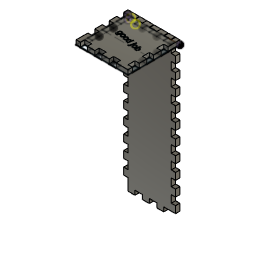
laser cut led  v7 (Autodesk Fusion 360 design; units mm, degrees)
Autodesk Fusion 360 part; units mm, degrees
sketch "Sketch1" plane through (0, 0, 0) normal (0, 1, 0) x (1, 0, 0)
  line L0 (0, 0) -> (30, 0)
  line L1 (30, 0) -> (30, -100)
  line L2 (30, -100) -> (0, -100)
  line L3 (0, -100) -> (0, 0)
  line L4 (0, 0) -> (4.8, 0)
  line L5 (4.8, 0) -> (4.8, 3)
  line L6 (4.8, 3) -> (0, 3)
  line L7 (0, 3) -> (0, 0)
  line L8 (4.8, 3) -> (10, 3) construction
  line L9 (10, 3) -> (14.8, 3)
  line L10 (14.8, 3) -> (14.8, 0)
  line L11 (14.8, 0) -> (10, 0)
  line L12 (10, 0) -> (10, 3)
  line L13 (14.8, 3) -> (20, 3) construction
  line L14 (20, 3) -> (24.8, 3)
  line L15 (24.8, 3) -> (24.8, 0)
  line L16 (24.8, 0) -> (20, 0)
  line L17 (20, 0) -> (20, 3)
  line L18 (0, -50) -> (30, -50) construction
  line L19 (30, 0) -> (33, 0)
  line L20 (33, 0) -> (33, -4.8)
  line L21 (33, -4.8) -> (30, -4.8)
  line L22 (30, -4.8) -> (30, 0)
  line L23 (33, -4.8) -> (33, -10) construction
  line L24 (33, -14.8) -> (30, -14.8)
  line L25 (30, -14.8) -> (30, -10)
  line L26 (33, -10) -> (33, -14.8)
  line L27 (30, -10) -> (33, -10)
  line L28 (33, -14.8) -> (33, -20) construction
  line L29 (33, -24.8) -> (30, -24.8)
  line L30 (30, -24.8) -> (30, -20)
  line L31 (33, -20) -> (33, -24.8)
  line L32 (30, -20) -> (33, -20)
  line L33 (33, -24.8) -> (33, -30) construction
  line L34 (33, -34.8) -> (30, -34.8)
  line L35 (30, -34.8) -> (30, -30)
  line L36 (33, -30) -> (33, -34.8)
  line L37 (30, -30) -> (33, -30)
  line L38 (33, -34.8) -> (33, -40) construction
  line L39 (33, -44.8) -> (30, -44.8)
  line L40 (30, -44.8) -> (30, -40)
  line L41 (33, -40) -> (33, -44.8)
  line L42 (30, -40) -> (33, -40)
  line L43 (33, -44.8) -> (33, -50) construction
  line L44 (33, -54.8) -> (30, -54.8)
  line L45 (30, -54.8) -> (30, -50)
  line L46 (33, -50) -> (33, -54.8)
  line L47 (30, -50) -> (33, -50)
  line L48 (33, -54.8) -> (33, -60) construction
  line L49 (33, -64.8) -> (30, -64.8)
  line L50 (30, -64.8) -> (30, -60)
  line L51 (33, -60) -> (33, -64.8)
  line L52 (30, -60) -> (33, -60)
  line L53 (33, -64.8) -> (33, -70) construction
  line L54 (33, -74.8) -> (30, -74.8)
  line L55 (30, -74.8) -> (30, -70)
  line L56 (33, -70) -> (33, -74.8)
  line L57 (30, -70) -> (33, -70)
  line L58 (33, -74.8) -> (33, -80) construction
  line L59 (33, -84.8) -> (30, -84.8)
  line L60 (30, -84.8) -> (30, -80)
  line L61 (33, -80) -> (33, -84.8)
  line L62 (30, -80) -> (33, -80)
  line L63 (33, -84.8) -> (33, -90) construction
  line L64 (33, -94.8) -> (30, -94.8)
  line L65 (30, -94.8) -> (30, -90)
  line L66 (33, -90) -> (33, -94.8)
  line L67 (30, -90) -> (33, -90)
  line L68 (33, -94.8) -> (33, -100) construction
  line L69 (-3, -100) -> (-3, -95.2)
  line L70 (-3, -95.2) -> (0, -95.2)
  line L71 (0, -95.2) -> (0, -100)
  line L72 (-3, -100) -> (0, -100)
  line L73 (-3, -95.2) -> (-3, -90) construction
  line L74 (0, -85.2) -> (0, -90)
  line L75 (-3, -85.2) -> (0, -85.2)
  line L76 (-3, -90) -> (-3, -85.2)
  line L77 (-3, -90) -> (0, -90)
  line L78 (-3, -85.2) -> (-3, -80) construction
  line L79 (0, -75.2) -> (0, -80)
  line L80 (-3, -75.2) -> (0, -75.2)
  line L81 (-3, -80) -> (-3, -75.2)
  line L82 (-3, -80) -> (0, -80)
  line L83 (-3, -75.2) -> (-3, -70) construction
  line L84 (0, -65.2) -> (0, -70)
  line L85 (-3, -65.2) -> (0, -65.2)
  line L86 (-3, -70) -> (-3, -65.2)
  line L87 (-3, -70) -> (0, -70)
  line L88 (-3, -65.2) -> (-3, -60) construction
  line L89 (0, -55.2) -> (0, -60)
  line L90 (-3, -55.2) -> (0, -55.2)
  line L91 (-3, -60) -> (-3, -55.2)
  line L92 (-3, -60) -> (0, -60)
  line L93 (-3, -55.2) -> (-3, -50) construction
  line L94 (0, -45.2) -> (0, -50)
  line L95 (-3, -45.2) -> (0, -45.2)
  line L96 (-3, -50) -> (-3, -45.2)
  line L97 (-3, -50) -> (0, -50)
  line L98 (-3, -45.2) -> (-3, -40) construction
  line L99 (0, -35.2) -> (0, -40)
  line L100 (-3, -35.2) -> (0, -35.2)
  line L101 (-3, -40) -> (-3, -35.2)
  line L102 (-3, -40) -> (0, -40)
  line L103 (-3, -35.2) -> (-3, -30) construction
  line L104 (0, -25.2) -> (0, -30)
  line L105 (-3, -25.2) -> (0, -25.2)
  line L106 (-3, -30) -> (-3, -25.2)
  line L107 (-3, -30) -> (0, -30)
  line L108 (-3, -25.2) -> (-3, -20) construction
  line L109 (0, -15.2) -> (0, -20)
  line L110 (-3, -15.2) -> (0, -15.2)
  line L111 (-3, -20) -> (-3, -15.2)
  line L112 (-3, -20) -> (0, -20)
  line L113 (-3, -15.2) -> (-3, -10) construction
  line L114 (0, -5.2) -> (0, -10)
  line L115 (-3, -5.2) -> (0, -5.2)
  line L116 (-3, -10) -> (-3, -5.2)
  line L117 (-3, -10) -> (0, -10)
  line L118 (-3, -5.2) -> (-3, 0) construction
  line L119 (30, -100) -> (25.2, -100)
  line L120 (25.2, -100) -> (25.2, -103)
  line L121 (25.2, -103) -> (30, -103)
  line L122 (30, -103) -> (30, -100)
  line L123 (25.2, -103) -> (20, -103) construction
  line L124 (15.2, -100) -> (15.2, -103)
  line L125 (15.2, -103) -> (10, -103) construction
  line L126 (20, -103) -> (20, -100)
  line L127 (15.2, -103) -> (20, -103)
  line L128 (20, -100) -> (15.2, -100)
  line L129 (5.2, -100) -> (5.2, -103)
  line L130 (5.2, -103) -> (0, -103) construction
  line L131 (10, -103) -> (10, -100)
  line L132 (5.2, -103) -> (10, -103)
  line L133 (10, -100) -> (5.2, -100)
  point P0 (0, -90)
  point P1 (0, -80)
  point P2 (0, -70)
  point P3 (0, -60)
  point P4 (0, -50)
  point P5 (0, -40)
  point P6 (0, -30)
  point P7 (0, -20)
  point P8 (0, -10)
  dimension "d1" = 30
  dimension "d2" = 100
  dimension "d8" = 4.8
  dimension "d9" = 3
  dimension "d12" = 4.8
  dimension "d13" = 3
  dimension "d15" = 5.2
  dimension "d16" = 5.2
  dimension "d17" = 4.8
  dimension "d18" = 3
  dimension "d20" = 3
  dimension "d21" = 4.8
  dimension "d22" = 5.2
  dimension "d25" = 0
  dimension "d26" = -90
  dimension "d27" = 3
  dimension "d28" = 4.8
  dimension "d29" = 5.2
  dimension "d32" = 0
  dimension "d33" = 90
  dimension "d34" = 4.8
  dimension "d35" = 3
  dimension "d36" = 5.2
  dimension "d40" = -20
  dimension "d41" = 0
  constraint horizontal L0
  constraint vertical L1
  constraint vertical L3
  constraint coincident L0.start L3.end
  constraint horizontal L4
  constraint vertical L5
  constraint horizontal L6
  constraint vertical L7
  constraint perpendicular L5 L8
  constraint horizontal L9
  constraint vertical L10
  constraint horizontal L11
  constraint vertical L12
  constraint coincident L5.end L6.start
  constraint perpendicular L10 L13
  constraint horizontal L14
  constraint vertical L15
  constraint horizontal L16
  constraint vertical L17
  constraint midpoint L3 P4
  constraint midpoint L1 L18.end
  constraint horizontal L19
  constraint vertical L20
  constraint horizontal L21
  constraint vertical L22
  constraint perpendicular L21 L23
  constraint vertical L69
  constraint horizontal L70
  constraint vertical L71
  constraint parallel L2 L64
  constraint equal L70 L72
  constraint coincident L2.end L3.start
  constraint perpendicular L70 L73
  constraint horizontal L119
  constraint vertical L120
  constraint horizontal L121
  constraint vertical L122
  constraint perpendicular L120 L123
  measures "d1" distance of L0.start L0.end
  measures "d2" distance of L0.start L2.end
  measures "d8" distance of L0.start L4.end
  measures "d9" distance of L0.start L6.end
  measures "d12" distance of L8.end L9.end
  measures "d13" distance of L8.end L11.end
  measures "d15" distance of L5.end L8.end
  measures "d16" distance of L9.end L13.end
  measures "d17" distance of L13.end L14.end
  measures "d18" distance of L13.end L16.end
  measures "d20" distance of L0.end L19.end
  measures "d21" distance of L0.end L21.end
  measures "d22" distance of L20.end L23.end
  measures "d27" distance of L2.end L69.start
  measures "d28" distance of L2.end L70.end
  measures "d29" distance of L69.end L73.end
  measures "d34" distance of L1.end L119.end
  measures "d35" distance of L1.end L121.end
  measures "d36" distance of L120.end L123.end
extrude "Extrude1" add sketch "Sketch1" along normal blind 3 makes body 1
sketch "Sketch2" plane through (0, 0, 100) normal (0, 0, 1) x (-1, 0, 0)
  line L0 (0, 0) -> (-5.2, 0) construction
  line L1 (0, -2) -> (0, 0) construction
  line L2 (3, -3) -> (-33, -3)
  line L3 (-33, -3) -> (-33, 33)
  line L4 (-33, 33) -> (3, 33)
  line L5 (3, 33) -> (3, -3)
  line L6 (3, 0) -> (0, 0)
  line L7 (0, 0) -> (0, 4.8)
  line L8 (0, 4.8) -> (3, 4.8)
  line L9 (3, 4.8) -> (3, 0)
  line L10 (0, 4.8) -> (0, 10) construction
  line L11 (3, 10) -> (0, 10)
  line L12 (0, 10) -> (0, 14.8)
  line L13 (0, 14.8) -> (3, 14.8)
  line L14 (0, 14.8) -> (0, 20) construction
  line L15 (3, 14.8) -> (3, 10)
  line L16 (3, 20) -> (0, 20)
  line L17 (0, 20) -> (0, 24.8)
  line L18 (0, 24.8) -> (3, 24.8)
  line L19 (0, 24.8) -> (0, 30) construction
  line L20 (3, 24.8) -> (3, 20)
  line L21 (0, 30) -> (-4.8, 30)
  line L22 (-4.8, 30) -> (-4.8, 33)
  line L23 (-4.8, 33) -> (0, 33)
  line L24 (0, 33) -> (0, 30)
  line L25 (-4.8, 30) -> (-10, 30) construction
  line L26 (-14.8, 33) -> (-10, 33)
  line L27 (-14.8, 30) -> (-20, 30) construction
  line L28 (-10, 30) -> (-14.8, 30)
  line L29 (-10, 33) -> (-10, 30)
  line L30 (-14.8, 30) -> (-14.8, 33)
  line L31 (-24.8, 33) -> (-20, 33)
  line L32 (-24.8, 30) -> (-30, 30) construction
  line L33 (-20, 30) -> (-24.8, 30)
  line L34 (-20, 33) -> (-20, 30)
  line L35 (-24.8, 30) -> (-24.8, 33)
  line L36 (-30, 30) -> (-33, 30)
  line L37 (-33, 30) -> (-33, 25.2)
  line L38 (-33, 25.2) -> (-30, 25.2)
  line L39 (-30, 25.2) -> (-30, 30)
  line L40 (-30, 25.2) -> (-30, 20) construction
  line L41 (-30, 15.2) -> (-30, 20)
  line L42 (-30, 20) -> (-33, 20)
  line L43 (-33, 15.2) -> (-30, 15.2)
  line L44 (-33, 20) -> (-33, 15.2)
  line L45 (-30, 15.2) -> (-30, 10) construction
  line L46 (-30, 5.2) -> (-30, 10)
  line L47 (-30, 10) -> (-33, 10)
  line L48 (-33, 5.2) -> (-30, 5.2)
  line L49 (-33, 10) -> (-33, 5.2)
  line L50 (-30, 5.2) -> (-30, 0) construction
  line L51 (3, 15) -> (-33, 15) construction
  line L52 (-10, 0) -> (-14.8, 0) construction
  line L53 (-14.8, 0) -> (-14.8, -3)
  line L54 (-14.8, 0) -> (-20, 0)
  line L55 (-24.8, 0) -> (-24.8, -3)
  line L56 (-4.8, 0) -> (-10, 0)
  line L57 (-4.8, 0) -> (-4.8, -3)
  line L58 (0, -3) -> (0, 0) construction
  line L59 (0, 0) -> (-4.8, 0) construction
  line L60 (-10, -3) -> (-10, 0)
  line L61 (-20, -3) -> (-20, 0)
  line L62 (-20, 0) -> (-24.8, 0) construction
  line L63 (-4.8, -3) -> (0, -3)
  line L64 (-24.8, -3) -> (-20, -3)
  line L65 (-14.8, -3) -> (-10, -3)
  line L66 (-24.8, 0) -> (-29.6, 0)
  line L67 (-29.6, 0) -> (-29.6, -3)
  line L68 (-29.6, -3) -> (-24.8, -3) construction
  line L69 (-24.8, -3) -> (-24.8, 0) construction
  point P0 (3, -3)
  point P1 (-33, -3)
  point P2 (0, 10)
  point P3 (0, 10)
  point P4 (0, 20)
  point P5 (0, 20)
  dimension "d44" = 36
  dimension "d51" = 3
  dimension "d52" = 4.8
  dimension "d53" = 5.2
  dimension "d56" = 0
  dimension "d57" = 20
  dimension "d75" = 4.8
  dimension "d76" = 3
  dimension "d77" = 5.2
  dimension "d80" = -20
  dimension "d81" = 0
  dimension "d84" = 36
  dimension "d85" = 3
  dimension "d86" = 4.8
  dimension "d87" = 5.2
  dimension "d90" = 0
  dimension "d91" = -20
  dimension "d108" = 33
  dimension "d109" = 4.8
  constraint horizontal L2
  constraint horizontal L4
  constraint vertical L5
  constraint coincident P0 L2.start
  constraint coincident P1 L2.end
  constraint horizontal L6
  constraint vertical L7
  constraint horizontal L8
  constraint vertical L9
  constraint coincident L5 L6.start
  constraint perpendicular L8 L10
  constraint coincident L0.start L1.end
  constraint horizontal L21
  constraint vertical L22
  constraint horizontal L23
  constraint vertical L24
  constraint perpendicular L22 L25
  constraint horizontal L36
  constraint vertical L37
  constraint horizontal L38
  constraint vertical L39
  constraint perpendicular L38 L40
  constraint midpoint L5 L51.start
  constraint midpoint L3 L51.end
  constraint symmetric L19.end L51 L0.start
  constraint symmetric L21.end L51 L56.start
  constraint symmetric L22.end L51 L57.end
  constraint symmetric L23.end L51 L58.start
  constraint symmetric L25.end L51 L52.start
  constraint symmetric L26.start L51 L53.end
  constraint symmetric L26.end L51 L60.start
  constraint symmetric L27.start L51 L52.end
  constraint symmetric L27.end L51 L54.end
  constraint symmetric L31.start L51 L55.end
  constraint symmetric L31.end L51 L61.start
  constraint symmetric L32.start L51 L55.start
  constraint horizontal L66
  constraint vertical L67
  constraint horizontal L68
  constraint vertical L69
  measures "d44" distance of P1 L3.end
  measures "d51" distance of L6.start L0.start
  measures "d52" distance of L6.start L8.end
  measures "d53" distance of L7.end P3
  measures "d75" distance of L19.end L21.end
  measures "d76" distance of L19.end L23.end
  measures "d77" distance of L21.end L25.end
  measures "d84" distance of L3.end L4.end
  measures "d85" distance of L32.end L36.end
  measures "d86" distance of L32.end L38.end
  measures "d87" distance of L38.end L40.end
  measures "d108" distance of L4 L50.end
  measures "d109" distance of L55.start L66.end
extrude "Extrude4" add sketch "Sketch2" along normal blind 3 separate body contours L2 L3 L4 L5 L6 L7 L8 L11 L12 L13 L16 L17 L18 L21 L22 L24 L28 L29 L30 L33 L34 L35 L36 L38 L39 L41 L42 L43 L46 L47 L48 L53 L54 L55 L56 L57 L60 L61 L63 L64 L65 L66 L67 | L2 L56 L57 L60 | L2 L53 L54 L61 | L2 L55 L66 L67 makes body 2
sketch "Sketch3" plane through (0, 0, 103) normal (0, 0, 1) x (-1, 0, 0)
  line L0 (-33, -3) -> (3, -3)
  line L1 (3, -3) -> (3, 0)
  line L2 (3, 0) -> (0, 0)
  line L3 (0, 0) -> (0, 4.8)
  line L4 (0, 4.8) -> (3, 4.8)
  line L5 (3, 4.8) -> (3, 10)
  line L6 (3, 10) -> (0, 10)
  line L7 (0, 10) -> (0, 14.8)
  line L8 (0, 14.8) -> (3, 14.8)
  line L9 (3, 14.8) -> (3, 20)
  line L10 (3, 20) -> (0, 20)
  line L11 (0, 20) -> (0, 24.8)
  line L12 (0, 24.8) -> (3, 24.8)
  line L13 (3, 24.8) -> (3, 33)
  line L14 (3, 33) -> (0, 33)
  line L15 (0, 33) -> (0, 30)
  line L16 (0, 30) -> (-4.8, 30)
  line L17 (-4.8, 30) -> (-4.8, 33)
  line L18 (-4.8, 33) -> (-10, 33)
  line L19 (-10, 33) -> (-10, 30)
  line L20 (-10, 30) -> (-14.8, 30)
  line L21 (-14.8, 30) -> (-14.8, 33)
  line L22 (-14.8, 33) -> (-20, 33)
  line L23 (-20, 33) -> (-20, 30)
  line L24 (-20, 30) -> (-24.8, 30)
  line L25 (-24.8, 30) -> (-24.8, 33)
  line L26 (-24.8, 33) -> (-33, 33)
  line L27 (-33, 33) -> (-33, 30)
  line L28 (-33, 30) -> (-30, 30)
  line L29 (-30, 30) -> (-30, 25.2)
  line L30 (-30, 25.2) -> (-33, 25.2)
  line L31 (-33, 25.2) -> (-33, 20)
  line L32 (-33, 20) -> (-30, 20)
  line L33 (-30, 20) -> (-30, 15.2)
  line L34 (-30, 15.2) -> (-33, 15.2)
  line L35 (-33, 15.2) -> (-33, 10)
  line L36 (-33, 10) -> (-30, 10)
  line L37 (-30, 10) -> (-30, 5.2)
  line L38 (-30, 5.2) -> (-33, 5.2)
  line L39 (-33, 5.2) -> (-33, -3)
  line L40 (-6.1133, 15.5844) -> (-20.7441, 18.8917) construction
  line L41 (-20.7441, 18.8917) -> (-21.8466, 14.0148) construction
  line L42 (-21.8466, 14.0148) -> (-7.2157, 10.7074) construction
  line L43 (-7.2157, 10.7074) -> (-6.1133, 15.5844) construction
  line L44 (-14.5311, 12.3611) -> (-17.9487, -2.7575) construction
  line L45 (-21.2953, 16.4532) -> (-33, 19.0991) construction
  dimension "d97" = 5
  dimension "d98" = 15
  dimension "d106" = 15.5
  dimension "d107" = 12
  text T0 "good job" font "Arial" height 5 align ink ink in box 0 x 0 at (-6.1133, 15.5844) x (-0.975389, 0.220489) y (-0.220489, -0.975389) spacing 1 kerned height is em
  constraint perpendicular L40 L41
  constraint parallel L40 L42
  constraint parallel L41 L43
  constraint midpoint L42 L44.start
  constraint perpendicular L42 L44
  constraint midpoint L41 L45.start
  constraint perpendicular L41 L45
  constraint coincident L35 L45.end
  measures "d97" distance of L40.start L42.end
  measures "d98" distance of L41.end L42.end
  measures "d106" distance of L44.start L44.end
  measures "d107" distance of L45.start L45.end
extrude "Extrude5" cut sketch "Sketch3" against normal blind 1 text T0 bodies 2
sketch "TOP_DXF" plane through (0, 0, 103) normal (0, 0, 1) x (-1, 0, 0)
  spline S0 degree 3 poles (-10.2517, 15.4704) (-10.0879, 15.4205) (-9.7707, 15.3239) (-9.5682, 15.0623) (-9.4702, 14.9358) knots 0 0 0 0 0.049993 0.096791 0.096791 0.096791 0.096791
  spline S1 degree 3 poles (-9.4702, 14.9358) (-9.4051, 14.7805) (-9.263, 14.4413) (-9.3289, 14.0777) (-9.3646, 13.8807) knots 0 0 0 0 0.049486 0.108074 0.108074 0.108074 0.108074
  spline S2 degree 3 poles (-9.3646, 13.8807) (-9.4225, 13.67) (-9.5289, 13.2826) (-9.8458, 13.0393) (-9.9903, 12.9283) knots 0 0 0 0 0.063477 0.116753 0.116753 0.116753 0.116753
  spline S3 degree 3 poles (-9.9903, 12.9283) (-10.1253, 12.8727) (-10.4018, 12.7588) (-10.6978, 12.804) (-10.8492, 12.8271) knots 0 0 0 0 0.042941 0.087955 0.087955 0.087955 0.087955
  spline S4 degree 3 poles (-10.8492, 12.8271) (-11.0107, 12.877) (-11.3256, 12.9742) (-11.5266, 13.2347) (-11.6245, 13.3615) knots 0 0 0 0 0.049367 0.096242 0.096242 0.096242 0.096242
  spline S5 degree 3 poles (-11.6245, 13.3615) (-11.6914, 13.514) (-11.8346, 13.8403) (-11.7742, 14.1928) (-11.7421, 14.3806) knots 0 0 0 0 0.048869 0.104602 0.104602 0.104602 0.104602
  spline S6 degree 3 poles (-11.7421, 14.3806) (-11.7059, 14.5272) (-11.6409, 14.791) (-11.4893, 15.0157) (-11.422, 15.1154) knots 0 0 0 0 0.044866 0.080708 0.080708 0.080708 0.080708
  spline S7 degree 3 poles (-11.422, 15.1154) (-11.3476, 15.1913) (-11.1982, 15.3434) (-10.9979, 15.4168) (-10.8975, 15.4537) knots 0 0 0 0 0.03145 0.063109 0.063109 0.063109 0.063109
  spline S8 degree 3 poles (-10.8975, 15.4537) (-10.7914, 15.4771) (-10.5773, 15.5245) (-10.3609, 15.4885) (-10.2517, 15.4704) knots 0 0 0 0 0.032274 0.065137 0.065137 0.065137 0.065137
  line L0 (-17.4905, 13.3773) -> (-16.7013, 16.8683)
  line L1 (-16.7013, 16.8683) -> (-16.3037, 16.7784)
  line L2 (-16.3037, 16.7784) -> (-16.3758, 16.4593)
  spline S9 degree 3 poles (-16.3758, 16.4593) (-16.2604, 16.5485) (-16.0264, 16.7294) (-15.7324, 16.6937) (-15.5835, 16.6756) knots 0 0 0 0 0.042007 0.085152 0.085152 0.085152 0.085152
  spline S10 degree 3 poles (-15.5835, 16.6756) (-15.4862, 16.6463) (-15.2916, 16.5877) (-15.1407, 16.4514) (-15.0651, 16.3833) knots 0 0 0 0 0.03006 0.060176 0.060176 0.060176 0.060176
  spline S11 degree 3 poles (-15.0651, 16.3833) (-14.9989, 16.303) (-14.8635, 16.1389) (-14.8066, 15.9337) (-14.7775, 15.8289) knots 0 0 0 0 0.030848 0.063081 0.063081 0.063081 0.063081
  spline S12 degree 3 poles (-14.7775, 15.8289) (-14.7608, 15.7139) (-14.7259, 15.4736) (-14.7703, 15.2348) (-14.7934, 15.1104) knots 0 0 0 0 0.034627 0.072303 0.072303 0.072303 0.072303
  spline S13 degree 3 poles (-14.7934, 15.1104) (-14.8254, 14.9899) (-14.8874, 14.7567) (-15.0138, 14.5513) (-15.075, 14.4519) knots 0 0 0 0 0.037159 0.071956 0.071956 0.071956 0.071956
  spline S14 degree 3 poles (-15.075, 14.4519) (-15.1428, 14.3663) (-15.2749, 14.1997) (-15.467, 14.109) (-15.5604, 14.0648) knots 0 0 0 0 0.03227 0.062841 0.062841 0.062841 0.062841
  spline S15 degree 3 poles (-15.5604, 14.0648) (-15.6584, 14.0366) (-15.8561, 13.9796) (-16.0594, 14.0118) (-16.162, 14.0281) knots 0 0 0 0 0.030177 0.060923 0.060923 0.060923 0.060923
  spline S16 degree 3 poles (-16.162, 14.0281) (-16.2343, 14.0481) (-16.3746, 14.0869) (-16.491, 14.1743) (-16.5474, 14.2166) knots 0 0 0 0 0.022293 0.043242 0.043242 0.043242 0.043242
  spline S17 degree 3 poles (-16.5474, 14.2166) (-16.5961, 14.2635) (-16.692, 14.3559) (-16.7517, 14.4749) (-16.7811, 14.5335) knots 0 0 0 0 0.020129 0.039633 0.039633 0.039633 0.039633
  line L3 (-16.7811, 14.5335) -> (-17.0642, 13.2809)
  line L4 (-17.0642, 13.2809) -> (-17.4905, 13.3773)
  line L5 (-19.9456, 13.9322) -> (-19.8331, 14.4299)
  line L6 (-19.8331, 14.4299) -> (-19.4045, 14.333)
  line L7 (-19.4045, 14.333) -> (-19.517, 13.8353)
  line L8 (-19.517, 13.8353) -> (-19.9456, 13.9322)
  spline S18 degree 3 poles (-20.8272, 17.861) (-20.6633, 17.8111) (-20.3462, 17.7145) (-20.1436, 17.4529) (-20.0457, 17.3264) knots 0 0 0 0 0.049993 0.096791 0.096791 0.096791 0.096791
  spline S19 degree 3 poles (-20.0457, 17.3264) (-19.9806, 17.1711) (-19.8384, 16.8319) (-19.9043, 16.4684) (-19.94, 16.2713) knots 0 0 0 0 0.049486 0.108074 0.108074 0.108074 0.108074
  spline S20 degree 3 poles (-19.94, 16.2713) (-19.9979, 16.0606) (-20.1044, 15.6732) (-20.4212, 15.4299) (-20.5658, 15.3189) knots 0 0 0 0 0.063477 0.116753 0.116753 0.116753 0.116753
  spline S21 degree 3 poles (-20.5658, 15.3189) (-20.7008, 15.2633) (-20.9773, 15.1494) (-21.2732, 15.1946) (-21.4247, 15.2177) knots 0 0 0 0 0.042941 0.087955 0.087955 0.087955 0.087955
  spline S22 degree 3 poles (-21.4247, 15.2177) (-21.5862, 15.2676) (-21.9011, 15.3648) (-22.102, 15.6253) (-22.1999, 15.7522) knots 0 0 0 0 0.049367 0.096242 0.096242 0.096242 0.096242
  spline S23 degree 3 poles (-22.1999, 15.7522) (-22.2668, 15.9046) (-22.41, 16.2309) (-22.3497, 16.5834) (-22.3175, 16.7712) knots 0 0 0 0 0.048869 0.104602 0.104602 0.104602 0.104602
  spline S24 degree 3 poles (-22.3175, 16.7712) (-22.2814, 16.9178) (-22.2163, 17.1816) (-22.0648, 17.4063) (-21.9975, 17.506) knots 0 0 0 0 0.044866 0.080708 0.080708 0.080708 0.080708
  spline S25 degree 3 poles (-21.9975, 17.506) (-21.923, 17.5819) (-21.7736, 17.734) (-21.5734, 17.8074) (-21.473, 17.8443) knots 0 0 0 0 0.03145 0.063109 0.063109 0.063109 0.063109
  spline S26 degree 3 poles (-21.473, 17.8443) (-21.3669, 17.8677) (-21.1527, 17.9151) (-20.9363, 17.8791) (-20.8272, 17.861) knots 0 0 0 0 0.032274 0.065137 0.065137 0.065137 0.065137
  spline S27 degree 3 poles (-18.8569, 18.184) (-18.7773, 18.2389) (-18.6061, 18.3571) (-18.3993, 18.3238) (-18.2887, 18.3059) knots 0 0 0 0 0.027951 0.060151 0.060151 0.060151 0.060151
  spline S28 degree 3 poles (-18.2887, 18.3059) (-18.2319, 18.2911) (-18.1192, 18.2619) (-18.0149, 18.2103) (-17.9631, 18.1847) knots 0 0 0 0 0.017555 0.034816 0.034816 0.034816 0.034816
  line L9 (-17.9631, 18.1847) -> (-18.1264, 17.8387)
  spline S29 degree 3 poles (-18.1264, 17.8387) (-18.1624, 17.857) (-18.2251, 17.8889) (-18.2925, 17.9091) (-18.3213, 17.9178) knots 0 0 0 0 0.012055 0.021068 0.021068 0.021068 0.021068
  spline S30 degree 3 poles (-18.3213, 17.9178) (-18.3621, 17.9241) (-18.4394, 17.9362) (-18.5052, 17.8946) (-18.5362, 17.875) knots 0 0 0 0 0.011929 0.022586 0.022586 0.022586 0.022586
  spline S31 degree 3 poles (-18.5362, 17.875) (-18.566, 17.8289) (-18.6486, 17.7011) (-18.6792, 17.5509) (-18.6988, 17.455) knots 0 0 0 0 0.016359 0.045367 0.045367 0.045367 0.045367
  line L10 (-18.6988, 17.455) -> (-19.2995, 14.7974)
  line L11 (-19.2995, 14.7974) -> (-19.7282, 14.8943)
  line L12 (-19.7282, 14.8943) -> (-19.1253, 17.5614)
  spline S32 degree 3 poles (-19.1253, 17.5614) (-19.0951, 17.6956) (-19.0444, 17.921) (-18.9109, 18.1082) (-18.8569, 18.184) knots 0 0 0 0 0.040708 0.068392 0.068392 0.068392 0.068392
  spline S33 degree 3 poles (-23.6109, 18.4903) (-23.4732, 18.4425) (-23.1968, 18.3468) (-23.061, 18.0876) (-22.9929, 17.9576) knots 0 0 0 0 0.042061 0.084388 0.084388 0.084388 0.084388
  line L13 (-22.9929, 17.9576) -> (-22.9214, 18.2743)
  line L14 (-22.9214, 18.2743) -> (-22.5237, 18.1844)
  line L15 (-22.5237, 18.1844) -> (-23.3128, 14.6934)
  line L16 (-23.3128, 14.6934) -> (-23.7415, 14.7903)
  line L17 (-23.7415, 14.7903) -> (-23.4599, 16.0357)
  spline S34 degree 3 poles (-23.4599, 16.0357) (-23.5784, 15.9581) (-23.8132, 15.8044) (-24.0919, 15.8361) (-24.2299, 15.8518) knots 0 0 0 0 0.041098 0.081422 0.081422 0.081422 0.081422
  spline S35 degree 3 poles (-24.2299, 15.8518) (-24.3056, 15.873) (-24.4562, 15.915) (-24.5858, 16.0023) (-24.6503, 16.0458) knots 0 0 0 0 0.023409 0.046571 0.046571 0.046571 0.046571
  spline S36 degree 3 poles (-24.6503, 16.0458) (-24.7087, 16.0948) (-24.8238, 16.1917) (-24.8973, 16.3229) (-24.9335, 16.3876) knots 0 0 0 0 0.022662 0.044716 0.044716 0.044716 0.044716
  spline S37 degree 3 poles (-24.9335, 16.3876) (-24.9626, 16.4584) (-25.023, 16.6057) (-25.0417, 16.7639) (-25.0514, 16.846) knots 0 0 0 0 0.022849 0.047529 0.047529 0.047529 0.047529
  spline S38 degree 3 poles (-25.0514, 16.846) (-25.055, 16.9335) (-25.0623, 17.1122) (-25.0285, 17.2879) (-25.0113, 17.3776) knots 0 0 0 0 0.026177 0.053469 0.053469 0.053469 0.053469
  spline S39 degree 3 poles (-25.0113, 17.3776) (-24.9582, 17.5741) (-24.8602, 17.9366) (-24.5876, 18.1926) (-24.4627, 18.3099) knots 0 0 0 0 0.059654 0.110074 0.110074 0.110074 0.110074
  spline S40 degree 3 poles (-24.4627, 18.3099) (-24.3281, 18.3882) (-24.0637, 18.5422) (-23.7601, 18.5074) (-23.6109, 18.4903) knots 0 0 0 0 0.045374 0.089175 0.089175 0.089175 0.089175
  spline S41 degree 3 poles (-12.964, 16.0835) (-12.8002, 16.0336) (-12.483, 15.9371) (-12.2805, 15.6754) (-12.1825, 15.5489) knots 0 0 0 0 0.049993 0.096791 0.096791 0.096791 0.096791
  spline S42 degree 3 poles (-12.1825, 15.5489) (-12.1175, 15.3936) (-11.9753, 15.0544) (-12.0412, 14.6909) (-12.0769, 14.4938) knots 0 0 0 0 0.049486 0.108074 0.108074 0.108074 0.108074
  spline S43 degree 3 poles (-12.0769, 14.4938) (-12.1348, 14.2831) (-12.2412, 13.8957) (-12.5581, 13.6524) (-12.7027, 13.5414) knots 0 0 0 0 0.063477 0.116753 0.116753 0.116753 0.116753
  spline S44 degree 3 poles (-12.7027, 13.5414) (-12.8377, 13.4858) (-13.1141, 13.3719) (-13.4101, 13.4171) (-13.5616, 13.4402) knots 0 0 0 0 0.042941 0.087955 0.087955 0.087955 0.087955
  spline S45 degree 3 poles (-13.5616, 13.4402) (-13.7231, 13.4901) (-14.0379, 13.5873) (-14.2389, 13.8478) (-14.3368, 13.9747) knots 0 0 0 0 0.049367 0.096242 0.096242 0.096242 0.096242
  spline S46 degree 3 poles (-14.3368, 13.9747) (-14.4037, 14.1271) (-14.5469, 14.4534) (-14.4865, 14.8059) (-14.4544, 14.9937) knots 0 0 0 0 0.048869 0.104602 0.104602 0.104602 0.104602
  spline S47 degree 3 poles (-14.4544, 14.9937) (-14.4182, 15.1403) (-14.3532, 15.4041) (-14.2016, 15.6288) (-14.1343, 15.7286) knots 0 0 0 0 0.044866 0.080708 0.080708 0.080708 0.080708
  spline S48 degree 3 poles (-14.1343, 15.7286) (-14.0599, 15.8044) (-13.9105, 15.9565) (-13.7103, 16.03) (-13.6098, 16.0668) knots 0 0 0 0 0.03145 0.063109 0.063109 0.063109 0.063109
  spline S49 degree 3 poles (-13.6098, 16.0668) (-13.5037, 16.0903) (-13.2896, 16.1376) (-13.0732, 16.1017) (-12.964, 16.0835) knots 0 0 0 0 0.032274 0.065137 0.065137 0.065137 0.065137
  spline S50 degree 3 poles (-7.2155, 15.8028) (-7.0772, 15.7655) (-6.8193, 15.6959) (-6.622, 15.5169) (-6.5305, 15.4339) knots 0 0 0 0 0.042255 0.078798 0.078798 0.078798 0.078798
  spline S51 degree 3 poles (-6.5305, 15.4339) (-6.4677, 15.336) (-6.3355, 15.1297) (-6.3778, 14.8873) (-6.4, 14.7599) knots 0 0 0 0 0.033654 0.070921 0.070921 0.070921 0.070921
  line L18 (-6.4, 14.7599) -> (-6.8027, 14.916)
  spline S52 degree 3 poles (-6.8027, 14.916) (-6.8004, 14.977) (-6.796, 15.0904) (-6.8565, 15.1858) (-6.8845, 15.2298) knots 0 0 0 0 0.017825 0.033118 0.033118 0.033118 0.033118
  spline S53 degree 3 poles (-6.8845, 15.2298) (-6.9381, 15.2784) (-7.0558, 15.3848) (-7.2097, 15.4254) (-7.2933, 15.4474) knots 0 0 0 0 0.021405 0.046918 0.046918 0.046918 0.046918
  spline S54 degree 3 poles (-7.2933, 15.4474) (-7.3839, 15.4652) (-7.5478, 15.4975) (-7.7081, 15.4524) (-7.7799, 15.4322) knots 0 0 0 0 0.02721 0.049279 0.049279 0.049279 0.049279
  spline S55 degree 3 poles (-7.7799, 15.4322) (-7.8398, 15.3989) (-7.9629, 15.3305) (-8.0365, 15.2102) (-8.0743, 15.1484) knots 0 0 0 0 0.020205 0.041523 0.041523 0.041523 0.041523
  spline S56 degree 3 poles (-8.0743, 15.1484) (-8.099, 15.0829) (-8.1656, 14.9063) (-8.2049, 14.7216) (-8.2296, 14.6053) knots 0 0 0 0 0.020963 0.056553 0.056553 0.056553 0.056553
  spline S57 degree 3 poles (-8.2296, 14.6053) (-8.1091, 14.6795) (-7.8705, 14.8265) (-7.5923, 14.7941) (-7.4547, 14.778) knots 0 0 0 0 0.041161 0.081492 0.081492 0.081492 0.081492
  spline S58 degree 3 poles (-7.4547, 14.778) (-7.2952, 14.7275) (-6.9854, 14.6293) (-6.8151, 14.3533) (-6.7325, 14.2193) knots 0 0 0 0 0.048395 0.094066 0.094066 0.094066 0.094066
  spline S59 degree 3 poles (-6.7325, 14.2193) (-6.6794, 14.0664) (-6.5702, 13.7513) (-6.6234, 13.4218) (-6.6507, 13.2522) knots 0 0 0 0 0.047772 0.098415 0.098415 0.098415 0.098415
  spline S60 degree 3 poles (-6.6507, 13.2522) (-6.6822, 13.1361) (-6.7437, 12.909) (-6.8706, 12.7108) (-6.9327, 12.6138) knots 0 0 0 0 0.035833 0.07015 0.07015 0.07015 0.07015
  spline S61 degree 3 poles (-6.9327, 12.6138) (-7.0016, 12.5292) (-7.1356, 12.3645) (-7.3266, 12.272) (-7.4194, 12.227) knots 0 0 0 0 0.032303 0.062844 0.062844 0.062844 0.062844
  spline S62 degree 3 poles (-7.4194, 12.227) (-7.5185, 12.1983) (-7.7231, 12.1392) (-7.9333, 12.1743) (-8.0416, 12.1925) knots 0 0 0 0 0.030558 0.063037 0.063037 0.063037 0.063037
  spline S63 degree 3 poles (-8.0416, 12.1925) (-8.1813, 12.2405) (-8.4635, 12.3377) (-8.6193, 12.5925) (-8.698, 12.7213) knots 0 0 0 0 0.042886 0.08668 0.08668 0.08668 0.08668
  line L19 (-8.698, 12.7213) -> (-8.7669, 12.4165)
  line L20 (-8.7669, 12.4165) -> (-9.1622, 12.5058)
  line L21 (-9.1622, 12.5058) -> (-8.6681, 14.6919)
  spline S64 degree 3 poles (-8.6681, 14.6919) (-8.6298, 14.8618) (-8.5654, 15.1474) (-8.4183, 15.3995) (-8.3586, 15.5017) knots 0 0 0 0 0.051819 0.087139 0.087139 0.087139 0.087139
  spline S65 degree 3 poles (-8.3586, 15.5017) (-8.294, 15.5695) (-8.1621, 15.708) (-7.9817, 15.7722) (-7.8896, 15.805) knots 0 0 0 0 0.027661 0.056549 0.056549 0.056549 0.056549
  spline S66 degree 3 poles (-7.8896, 15.805) (-7.7846, 15.825) (-7.5601, 15.8678) (-7.3352, 15.8254) (-7.2155, 15.8028) knots 0 0 0 0 0.031775 0.067941 0.067941 0.067941 0.067941
  line L22 (-33, -3) -> (3, -3)
  line L23 (3, -3) -> (3, 0)
  line L24 (3, 0) -> (0, 0)
  line L25 (0, 0) -> (0, 4.8)
  line L26 (0, 4.8) -> (3, 4.8)
  line L27 (3, 4.8) -> (3, 10)
  line L28 (3, 10) -> (0, 10)
  line L29 (0, 10) -> (0, 14.8)
  line L30 (0, 14.8) -> (3, 14.8)
  line L31 (3, 14.8) -> (3, 20)
  line L32 (3, 20) -> (0, 20)
  line L33 (0, 20) -> (0, 24.8)
  line L34 (0, 24.8) -> (3, 24.8)
  line L35 (3, 24.8) -> (3, 33)
  line L36 (3, 33) -> (0, 33)
  line L37 (0, 33) -> (0, 30)
  line L38 (0, 30) -> (-4.8, 30)
  line L39 (-4.8, 30) -> (-4.8, 33)
  line L40 (-4.8, 33) -> (-10, 33)
  line L41 (-10, 33) -> (-10, 30)
  line L42 (-10, 30) -> (-14.8, 30)
  line L43 (-14.8, 30) -> (-14.8, 33)
  line L44 (-14.8, 33) -> (-20, 33)
  line L45 (-20, 33) -> (-20, 30)
  line L46 (-20, 30) -> (-24.8, 30)
  line L47 (-24.8, 30) -> (-24.8, 33)
  line L48 (-24.8, 33) -> (-33, 33)
  line L49 (-33, 33) -> (-33, 30)
  line L50 (-33, 30) -> (-30, 30)
  line L51 (-30, 30) -> (-30, 25.2)
  line L52 (-30, 25.2) -> (-33, 25.2)
  line L53 (-33, 25.2) -> (-33, 20)
  line L54 (-33, 20) -> (-30, 20)
  line L55 (-30, 20) -> (-30, 15.2)
  line L56 (-30, 15.2) -> (-33, 15.2)
  line L57 (-33, 15.2) -> (-33, 10)
  line L58 (-33, 10) -> (-30, 10)
  line L59 (-30, 10) -> (-30, 5.2)
  line L60 (-30, 5.2) -> (-33, 5.2)
  line L61 (-33, 5.2) -> (-33, -3)
sketch "4Sides_DXF" plane through (0, 3, 0) normal (0, 1, 0) x (-1, 0, 0)
  line L0 (-5.2, 100) -> (-5.2, 103)
  line L1 (-5.2, 103) -> (-10, 103)
  line L2 (-10, 103) -> (-10, 100)
  line L3 (-10, 100) -> (-15.2, 100)
  line L4 (-15.2, 100) -> (-15.2, 103)
  line L5 (-15.2, 103) -> (-20, 103)
  line L6 (-20, 103) -> (-20, 100)
  line L7 (-20, 100) -> (-25.2, 100)
  line L8 (-25.2, 100) -> (-25.2, 103)
  line L9 (-25.2, 103) -> (-30, 103)
  line L10 (-30, 103) -> (-30, 94.8)
  line L11 (-30, 94.8) -> (-33, 94.8)
  line L12 (-33, 94.8) -> (-33, 90)
  line L13 (-33, 90) -> (-30, 90)
  line L14 (-30, 90) -> (-30, 84.8)
  line L15 (-30, 84.8) -> (-33, 84.8)
  line L16 (-33, 84.8) -> (-33, 80)
  line L17 (-33, 80) -> (-30, 80)
  line L18 (-30, 80) -> (-30, 74.8)
  line L19 (-30, 74.8) -> (-33, 74.8)
  line L20 (-33, 74.8) -> (-33, 70)
  line L21 (-33, 70) -> (-30, 70)
  line L22 (-30, 70) -> (-30, 64.8)
  line L23 (-30, 64.8) -> (-33, 64.8)
  line L24 (-33, 64.8) -> (-33, 60)
  line L25 (-33, 60) -> (-30, 60)
  line L26 (-30, 60) -> (-30, 54.8)
  line L27 (-30, 54.8) -> (-33, 54.8)
  line L28 (-33, 54.8) -> (-33, 50)
  line L29 (-33, 50) -> (-30, 50)
  line L30 (-30, 50) -> (-30, 44.8)
  line L31 (-30, 44.8) -> (-33, 44.8)
  line L32 (-33, 44.8) -> (-33, 40)
  line L33 (-33, 40) -> (-30, 40)
  line L34 (-30, 40) -> (-30, 34.8)
  line L35 (-30, 34.8) -> (-33, 34.8)
  line L36 (-33, 34.8) -> (-33, 30)
  line L37 (-33, 30) -> (-30, 30)
  line L38 (-30, 30) -> (-30, 24.8)
  line L39 (-30, 24.8) -> (-33, 24.8)
  line L40 (-33, 24.8) -> (-33, 20)
  line L41 (-33, 20) -> (-30, 20)
  line L42 (-30, 20) -> (-30, 14.8)
  line L43 (-30, 14.8) -> (-33, 14.8)
  line L44 (-33, 14.8) -> (-33, 10)
  line L45 (-33, 10) -> (-30, 10)
  line L46 (-30, 10) -> (-30, 4.8)
  line L47 (-30, 4.8) -> (-33, 4.8)
  line L48 (-33, 4.8) -> (-33, 0)
  line L49 (-33, 0) -> (-24.8, 0)
  line L50 (-24.8, 0) -> (-24.8, -3)
  line L51 (-24.8, -3) -> (-20, -3)
  line L52 (-20, -3) -> (-20, 0)
  line L53 (-20, 0) -> (-14.8, 0)
  line L54 (-14.8, 0) -> (-14.8, -3)
  line L55 (-14.8, -3) -> (-10, -3)
  line L56 (-10, -3) -> (-10, 0)
  line L57 (-10, 0) -> (-4.8, 0)
  line L58 (-4.8, 0) -> (-4.8, -3)
  line L59 (-4.8, -3) -> (0, -3)
  line L60 (0, -3) -> (0, 5.2)
  line L61 (0, 5.2) -> (3, 5.2)
  line L62 (3, 5.2) -> (3, 10)
  line L63 (3, 10) -> (0, 10)
  line L64 (0, 10) -> (0, 15.2)
  line L65 (0, 15.2) -> (3, 15.2)
  line L66 (3, 15.2) -> (3, 20)
  line L67 (3, 20) -> (0, 20)
  line L68 (0, 20) -> (0, 25.2)
  line L69 (0, 25.2) -> (3, 25.2)
  line L70 (3, 25.2) -> (3, 30)
  line L71 (3, 30) -> (0, 30)
  line L72 (0, 30) -> (0, 35.2)
  line L73 (0, 35.2) -> (3, 35.2)
  line L74 (3, 35.2) -> (3, 40)
  line L75 (3, 40) -> (0, 40)
  line L76 (0, 40) -> (0, 45.2)
  line L77 (0, 45.2) -> (3, 45.2)
  line L78 (3, 45.2) -> (3, 50)
  line L79 (3, 50) -> (0, 50)
  line L80 (0, 50) -> (0, 55.2)
  line L81 (0, 55.2) -> (3, 55.2)
  line L82 (3, 55.2) -> (3, 60)
  line L83 (3, 60) -> (0, 60)
  line L84 (0, 60) -> (0, 65.2)
  line L85 (0, 65.2) -> (3, 65.2)
  line L86 (3, 65.2) -> (3, 70)
  line L87 (3, 70) -> (0, 70)
  line L88 (0, 70) -> (0, 75.2)
  line L89 (0, 75.2) -> (3, 75.2)
  line L90 (3, 75.2) -> (3, 80)
  line L91 (3, 80) -> (0, 80)
  line L92 (0, 80) -> (0, 85.2)
  line L93 (0, 85.2) -> (3, 85.2)
  line L94 (3, 85.2) -> (3, 90)
  line L95 (3, 90) -> (0, 90)
  line L96 (0, 90) -> (0, 95.2)
  line L97 (0, 95.2) -> (3, 95.2)
  line L98 (3, 95.2) -> (3, 100)
  line L99 (3, 100) -> (-5.2, 100)
extrude "Extrude6" cut sketch "Sketch2" along normal up to surface (3 mm away) contours L2 L56 L57 L60 | L2 L53 L54 L61 | L2 L55 L66 L67 bodies 2
equation "d1 = br"
equation "d2 = le"
equation "de = 3 mm"
equation "sbr = 4.8 mm"
equation "le = 100 mm"
equation "br = 30 mm"
equation "wi = br"
equation "d8 = sbr"
equation "d9 = de"
equation "d12 = sbr"
equation "d13 = de"
equation "sbre = 5.2 mm"
equation "d15 = sbre"
equation "d16 = sbre"
equation "d17 = sbr"
equation "d18 = de"
equation "lesbr = le / ( sbr + sbre )"
equation "d20 = de"
equation "d21 = sbr"
equation "d22 = sbre"
equation "d24 = lesbr"
equation "d27 = de"
equation "d28 = sbr"
equation "d29 = sbre"
equation "d31 = lesbr"
equation "d34 = sbr"
equation "d35 = de"
equation "d36 = sbre"
equation "bwsbr = br / ( sbr + sbre )"
equation "d38 = bwsbr"
equation "d40 = -30 mm + 10 mm"
equation "d42 = de"
equation "d44 = de * 2 + br"
equation "d51 = de"
equation "d52 = sbr"
equation "d53 = sbre"
equation "d55 = bwsbr"
equation "d57 = 30 mm - 10 mm"
equation "d75 = sbr"
equation "d76 = de"
equation "d77 = sbre"
equation "d78 = bwsbr"
equation "d80 = -30 mm + 10 mm"
equation "d85 = de"
equation "d86 = sbr"
equation "d87 = sbre"
equation "d89 = bwsbr"
equation "d91 = -( 30 mm - 10 mm )"
equation "d92 = de"
equation "txth = 5 mm"
equation "txtl = br / 2"
equation "d97 = txth"
equation "d98 = txtl"
equation "txtls = ( br + de * 2 - txtl ) / 2 + 1.5 mm"
equation "txths = ( wi + de * 2 - txth ) / 2"
equation "d106 = txths"
equation "d107 = txtls"
named bodies: "LaserCut"
